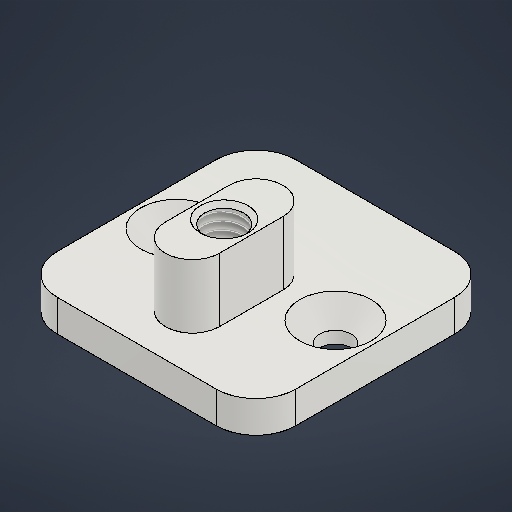
# Autodesk Inventor part: TCSM1-004
Saved by Autodesk Inventor 2025.3 (Build 293356000, 356)
## iProperties
Created: 2025-08-26
Part Number: TCSM1-004
Material: Steel
Document SubType Name: Modeling
Designer: fablabadmin
Density: 7.85 g/cm^3
Appearance: Steel
Author: fablabadmin
Autodesk Inventor part; units mm, degrees
ref_plane "YZ Plane" through (0, 0, 0) normal (1, 0, 0) x (0, 1, 0)
ref_plane "XZ Plane" through (0, 0, 0) normal (0, 1, 0) x (-1, 0, 0)
ref_plane "XY Plane" through (0, 0, 0) normal (0, 0, 1) x (1, 0, 0)
sketch "Sketch1" plane through (0, 0, 0) normal (0, 1, 0) x (-1, 0, 0)
  line L0 (-15, 15) -> (15, 15)
  line L1 (15, 15) -> (15, -15)
  line L2 (15, -15) -> (-15, -15)
  line L3 (-15, -15) -> (-15, 15)
  line L4 (-15, 15) -> (15, -15) construction
  line L5 (15, 15) -> (-15, -15) construction
  line L6 (21, 0) -> (-21, 0) construction
  line L7 (0, -21) -> (0, 21) construction
  line L8 (0, 8) -> (0, 0) construction
  line L9 (-3.4, 8) -> (-3.4, 0)
  line L10 (3.4, 0) -> (3.4, 8)
  arc A0 (3.4, 8) -> (-3.4, 8) centre (0, 8) ccw
  arc A1 (-3.4, 0) -> (3.4, 0) centre (0, 0) ccw
  point P0 (0, 0)
  point P1 (0, 4)
  point P2 (10, 0)
  point P3 (-10, 0)
  point P4 (0, 4)
  dimension "d0" = 30
  dimension "d1" = 30
  dimension "d2" = 6.8
  dimension "d3" = 8
  dimension "d4" = 0
  dimension "d5" = 20
  constraints: 20 end point, 4 midpoint, 4 point on circle, 4 tangent, 3 parallel, 2 centre point, 2 point on line, 1 coincident, 1 horizontal, 1 perpendicular, 1 symmetric about line
  measures "d0" distance of L0.start L0.end
  measures "d1" distance of L0.end L1.end
  measures "d2" distance between parallel lines of L9 L10
  measures "d3" distance of L8.end L8.start
  measures "d4" distance of point (0, 0) L8.end
  measures "d5" distance of point (-10, 0) point (10, 0)
extrude "Extrusion1" add sketch "Sketch1" against normal blind 12 contours L0 L1 L2 L3 | A0 L10 A1 L9
extrude "Extrusion2" cut sketch "Sketch1" against normal blind 8
hole "Hole1" at (0, 0, 4) direction (0, -1, 0) diameter 4.917 end through all countersink diameter 6 countersink angle 90 thread size "M6x1" class "6H" standard "ISO Metric profile"
sketch "Sketch2" plane through (0, -8, 0) normal (0, 1, 0) x (1, 0, 0)
  point P0 (0, 0)
  point P1 (10, 0)
  point P2 (-10, 0)
hole "Hole2" at (10, -8, 0) at (-10, -8, 0) direction (0, -1, 0) diameter 4 end through all countersink diameter 9 countersink angle 90
fillet "Fillet1" radius 5 4 edges at (-15, -10, -15) (-15, -10, 15) (15, -10, 15) (15, -10, -15)
body "Solid1"
